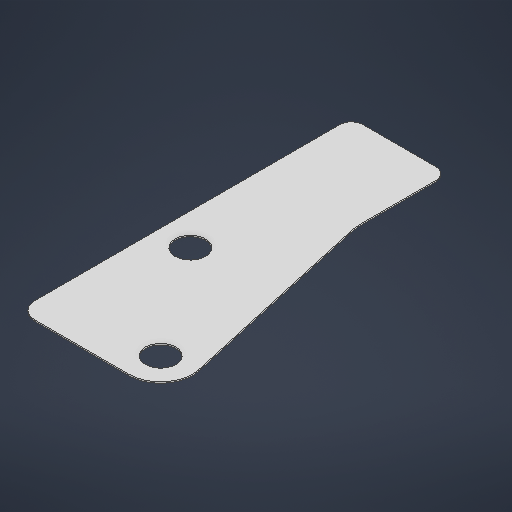
# Autodesk Inventor part: core_housing_master
Saved by Autodesk Inventor 2026 (Build 300175000, 175)
## iProperties
Created: 2025-05-09
Part Number: core_housing_master
Material: Generic
Document SubType Name: Modeling
Designer: Paul Juschitz
Density: 1 g/cm^3
Appearance: Default
d0: 1,000 ul
d1: 1,000 ul
d2: 151,500 mm
d3: 14,300 mm
d4: 5,000 ul
d8: 54,000 mm
d9: 5,000 mm
d10: 2,000 mm
core_housing_foot_outer_spacing: 10,000 mm
d16: 10,000 mm
core_housing_foot_inner_spacing: 2,000 mm
d18: 2,000 mm
d19: 0,800 mm
d20: 0,00 deg
core_housing_tolerance: 0,200 mm
core_housing_material_thickness: 0,800 mm
d6: 360,00 deg
m2m_bottom_cover_diameter: 151,500 mm
m2m_bottom_foot_diameter: 14,300 mm
core_outer_width: 54,000 mm
core_outer_radius: 5,000 mm
core_height: 25,000 mm
core_inner_width: 50,400 mm
Author: Paul Juschitz
Autodesk Inventor part; units mm, degrees
ref_plane "YZ Plane" through (0, 0, 0) normal (1, 0, 0) x (0, 1, 0)
ref_plane "XZ Plane" through (0, 0, 0) normal (0, 1, 0) x (-1, 0, 0)
ref_plane "XY Plane" through (0, 0, 0) normal (0, 0, 1) x (1, 0, 0)
derived "m2m_bottom_2.ipt"
derived "core_dummy_1.ipt"
sketch "Sketch1" plane through (0, 0, 0) normal (0, 1, 0) x (-1, 0, 0)
  circle A0 centre (0, 0) radius 75.75 construction
  circle A1 centre (55.4986, -40.3221) radius 7.15 construction
  circle A2 centre (55.4986, 40.3221) radius 7.15 construction
  circle A3 centre (-21.1986, 65.2425) radius 7.15 construction
  circle A4 centre (-68.6, 0) radius 7.15 construction
  circle A5 centre (-21.1986, -65.2425) radius 7.15 construction
  line L0 (-9.0486, -125.2425) -> (-53.0486, -125.2425) construction
  line L1 (-58.0486, -130.2425) -> (-58.0486, -174.2425) construction
  line L2 (-53.0486, -179.2425) -> (-9.0486, -179.2425) construction
  line L3 (-4.0486, -174.2425) -> (-4.0486, -130.2425) construction
  arc A6 (-4.0486, -130.2425) -> (-9.0486, -125.2425) centre (-9.0486, -130.2425) ccw construction
  arc A7 (-9.0486, -179.2425) -> (-4.0486, -174.2425) centre (-9.0486, -174.2425) ccw construction
  arc A8 (-58.0486, -174.2425) -> (-53.0486, -179.2425) centre (-53.0486, -174.2425) ccw construction
  arc A9 (-53.0486, -125.2425) -> (-58.0486, -130.2425) centre (-53.0486, -130.2425) ccw construction
  line L4 (-53.0486, -123.2425) -> (-9.0486, -123.2425) construction
  arc A10 (-2.0486, -130.2425) -> (-9.0486, -123.2425) centre (-9.0486, -130.2425) ccw construction
  line L5 (-2.0486, -130.2425) -> (-2.0486, -174.2425)
  arc A11 (-9.0486, -181.2425) -> (-2.0486, -174.2425) centre (-9.0486, -174.2425) ccw
  line L6 (-9.0486, -181.2425) -> (-53.0486, -181.2425)
  arc A12 (-60.0486, -174.2425) -> (-53.0486, -181.2425) centre (-53.0486, -174.2425) ccw
  line L7 (-60.0486, -174.2425) -> (-60.0486, -130.2425)
  arc A13 (-53.0486, -123.2425) -> (-60.0486, -130.2425) centre (-53.0486, -130.2425) ccw construction
  arc A14 (-68.6, 19.15) -> (-87.2872, -4.1848) centre (-68.6, 0) ccw
  line L8 (-68.6, 19.15) -> (-12.0486, 19.15)
  line L9 (-2.0486, 9.15) -> (-2.0486, -65.2425)
  arc A15 (-2.0486, -65.2425) -> (-2.0486, -65.2425) centre (-21.1986, -65.2425) ccw
  line L10 (-2.0486, -65.2425) -> (-2.0486, -130.2425)
  arc A16 (-2.0486, -130.2425) -> (-2.0486, -130.2425) centre (17.1014, -130.2425) ccw
  arc A17 (-2.0486, 9.15) -> (-12.0486, 19.15) centre (-12.0486, 9.15) ccw
  circle A18 centre (-21.1986, -65.2425) radius 9.15
  circle A19 centre (-68.6, 0) radius 9.15
  line L11 (-87.2872, -4.1848) -> (-61.0153, -121.5014)
  arc A20 (-60.0486, -130.2425) -> (-61.0153, -121.5014) centre (-100.0486, -130.2425) ccw
  point P0 (-58.0486, -179.2425)
  point P1 (-58.0486, -125.2425)
  dimension "d2" = 151.5
  dimension "d3" = 14.3
  dimension "d6" = 360
  dimension "d8" = 54
  dimension "d9" = 5
  dimension "d10" = 2
  dimension "d16" = 10
  dimension "core_housing_foot_inner_spacing" = 2
  dimension "d18" = 2
  dimension "d21" = 10
  dimension "d22" = 10
  dimension "d23" = 65
  dimension "d24" = 40
  constraints: 26 point on circle, 24 end point, 21 centre point, 19 tangent, 4 equal radius, 4 parallel, 4 perpendicular, 4 point on line, 2 concentric, 2 vertical, 1 coincident, 1 horizontal, 1 horizontal alignment, 18 other
  measures "d2" diameter of A0
  measures "d3" diameter of A1
  measures "d8" distance of point (-58.049, -125.242) point (-58.049, -179.242)
  measures "d9" radius of A6
  measures "d10" distance between parallel lines of L0 L4
  measures "d16" radius of A17
  measures "core_housing_foot_inner_spacing" radial gap between concentric circles of A5 A18
  measures "d18" radial gap between concentric circles of A4 A19
  measures "d21" radial gap between concentric circles of A19 A14
  measures "d22" radial gap between concentric circles of A18 A15
  measures "d23" distance of L10.start L10.end
  measures "d24" radius of A20
extrude "Extrusion2" add sketch "Sketch1" along normal blind 0.8 contours A15 | L5 A11 L6 A12 L7 A20 L11 A14 L8 A17 L9 L10
equation "\"d2\" = m2m_bottom_cover_diameter"
equation "\"d3\" = m2m_bottom_foot_diameter"
equation "\"d8\" = core_outer_width"
equation "\"d9\" = core_outer_radius"
equation "\"d10\" = 2 * core_housing_material_thickness + 2 * core_housing_tolerance"
equation "\"d16\" = core_housing_foot_outer_spacing"
equation "\"d18\" = core_housing_foot_inner_spacing"
equation "\"d19\" = core_housing_material_thickness"
equation "\"core_housing_tolerance\" = 0.2"
equation "\"core_housing_material_thickness\" = 0.8"
equation "\"m2m_bottom_cover_diameter\" = 151.5"
equation "\"m2m_bottom_foot_diameter\" = 14.3"
equation "\"core_outer_radius\" = 5"
equation "\"core_housing_foot_outer_spacing\" = 10"
equation "\"core_outer_width\" = 54"
body "Solid2"
